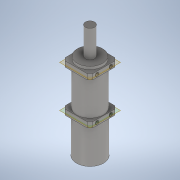
# Autodesk Inventor part: Motor
Saved by Autodesk Inventor 2022 (Build 260153000, 153)
## iProperties
Created: 2021-10-22
Part Number: Motor
Material: Stainless Steel
Document SubType Name: Modeling
Designer: juanp
Density: 8 g/cm^3
Appearance: Semi-Polished
Author: juanp
Autodesk Inventor part; units mm, degrees
ref_plane "YZ Plane" through (0, 0, 0) normal (1, 0, 0) x (0, 1, 0)
ref_plane "XZ Plane" through (0, 0, 0) normal (0, 1, 0) x (-1, 0, 0)
ref_plane "XY Plane" through (0, 0, 0) normal (0, 0, 1) x (1, 0, 0)
sketch "Sketch1" plane through (0, 0, 0) normal (0, 1, 0) x (-1, 0, 0)
  circle A0 centre (0, 0) radius 18.675
  dimension "d0" = 37.35
  constraints: 1 centre point, 1 coincident
  measures "d0" diameter of A0
extrude "Extrusion1" add sketch "Sketch1" along normal blind 50
sketch "Sketch2" plane through (0, 50, 0) normal (0, 1, 0) x (1, 0, 0)
  line L0 (-19.125, -19.125) -> (19.125, -19.125)
  line L1 (19.125, -19.125) -> (19.125, 19.125)
  line L2 (19.125, 19.125) -> (-19.125, 19.125)
  line L3 (-19.125, 19.125) -> (-19.125, -19.125)
  line L4 (-19.125, -19.125) -> (19.125, 19.125) construction
  line L5 (19.125, -19.125) -> (-19.125, 19.125) construction
  point P0 (0, 0)
  dimension "d3" = 38.25
  constraints: 12 end point, 2 midpoint, 2 parallel, 2 perpendicular, 1 horizontal
  measures "d3" distance of L2.end L0.start
extrude "Extrusion2" add sketch "Sketch2" along normal blind 7.5
chamfer "Chamfer1" distance 4 angle 45 4 edges at (-19.125, 53.75, -19.125) (-19.125, 53.75, 19.125) (19.125, 53.75, 19.125) (19.125, 53.75, -19.125)
sketch "Sketch3" plane through (0, 57.5, 0) normal (0, 1, 0) x (1, 0, 0)
  circle A0 centre (0, 0) radius 18.4
  dimension "d9" = 36.8
  constraints: 1 centre point, 1 coincident
  measures "d9" diameter of A0
extrude "Extrusion3" add sketch "Sketch3" along normal blind 50
ref_plane "Work Plane1" through (0, 82.5, 0) normal (0, 1, 0) x (1, 0, 0)
mirror "Mirror1" about plane through (0, 82.5, 0) normal (0, 1, 0) of "Extrusion2", "Chamfer1"
sketch "Sketch4" plane through (-15.125, 115, -19.125) normal (0, 1, 0) x (1, 0, 0)
  circle A0 centre (15.125, -19.125) radius 17.5
  dimension "d12" = 35
  constraints: 1 centre point, 1 coincident
  measures "d12" diameter of A0
extrude "Extrusion4" add sketch "Sketch4" along normal blind 3.85
sketch "Sketch5" plane through (0, 118.85, 0) normal (0, 1, 0) x (1, 0, 0)
  circle A0 centre (0, 0) radius 6.35
  dimension "d15" = 12.7
  constraints: 1 centre point, 1 coincident
  measures "d15" diameter of A0
extrude "Extrusion5" add sketch "Sketch5" along normal blind 37.6
sketch "Sketch6" plane through (19.125, 115, 15.125) normal (1, 0, 0) x (0, 0, -1)
  line L0 (30.25, -7.5) -> (30.25, 0) construction
  line L1 (0, 0) -> (30.25, 0) construction
  line L2 (0, 0) -> (0, -7.5) construction
  line L3 (0, -7.5) -> (30.25, -7.5) construction
  line L4 (30.25, -57.5) -> (30.25, -65) construction
  line L5 (0, -57.5) -> (30.25, -57.5) construction
  line L6 (0, -65) -> (0, -57.5) construction
  line L7 (0, -65) -> (30.25, -65) construction
  line L8 (0, -3.75) -> (5.6, -3.75) construction
  line L9 (5.6, -3.75) -> (24.65, -3.75) construction
  line L10 (24.65, -3.75) -> (30.25, -3.75) construction
  line L11 (0, -57.5) -> (0, -65) projected
  line L12 (0, -61.25) -> (5.6, -61.25) construction
  line L13 (5.6, -61.25) -> (24.65, -61.25) construction
  line L14 (24.65, -61.25) -> (30.25, -61.25) construction
  circle A0 centre (5.6, -3.75) radius 2.4
  circle A1 centre (24.65, -3.75) radius 2.4
  circle A2 centre (5.6, -61.25) radius 2.4
  circle A3 centre (24.65, -61.25) radius 2.4
  point P0 (15.125, -115)
  dimension "d18" = 19.05
  dimension "d19" = 4.8
  constraints: 12 end point, 4 centre point, 4 coincident, 4 midpoint, 3 equal length, 3 equal radius, 2 horizontal, 2 point on line
  measures "d18" distance of L8.end L9.end
  measures "d19" diameter of A1
extrude "Extrusion6" cut sketch "Sketch6" against normal blind 10
mirror "Mirror2" about plane through (0, 0, 0) normal (1, 0, 0) of "Extrusion6"
ref_plane "Work Plane2" through (0, 137.65, 0) normal (0, 1, 0) x (1, 0, 0)
ref_plane "Work Plane3" through (-15.125, 111.25, -19.125) normal (0, 1, 0) x (1, 0, 0)
ref_plane "Work Plane4" through (0, 53.75, 0) normal (0, -1, 0) x (1, 0, 0)
body "Solid1"
